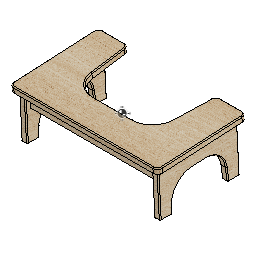
model (Autodesk Fusion 360 design; units mm, degrees)
Autodesk Fusion 360 part; units mm, degrees
sketch "top" plane through (0, 0, 0) normal (0, 0, 1) x (1, 0, 0) in component "stool"
  line L0 (0, 0) -> (500, 0)
  line L1 (120, 100.7611) -> (102.5689, 300)
  line L2 (102.5689, 300) -> (0, 300)
  line L3 (0, 300) -> (0, 0)
  line L4 (120, 100.7611) -> (380, 100.7611)
  line L5 (500, 300) -> (500, 0)
  line L6 (380, 100.7611) -> (397.4311, 300)
  line L7 (397.4311, 300) -> (500, 300)
  arc A0 (315.8568, 100.7611) -> (385.5904, 164.6602) centre (315.8568, 170.7611) ccw
  arc A1 (114.4096, 164.6602) -> (184.1432, 100.7611) centre (184.1432, 170.7611) ccw
  dimension "d5" = 300
  dimension "d6" = 500
  dimension "d7" = 260
  dimension "d8" = 200
  dimension "d21" = 70
  dimension "d36" = 95
  dimension "d37" = 95
  dimension "d42" = 294.8623
  dimension "d43" = 102.5689
  dimension "d44" = 100.7611
  constraint horizontal L0
  constraint horizontal L2
  constraint vertical L3
  constraint coincident L0.start L3.end
  constraint horizontal L4
  constraint vertical L5
  constraint horizontal L7
  constraint equal L2 L7
  constraint equal L3 L5
  constraint tangent L4 A0
  constraint coincident L4 A0.start
  constraint coincident L6 A0.end
  constraint tangent L1 A1
  constraint coincident L1 A1.start
  constraint coincident L4 A1.end
  constraint tangent L6 A0
  constraint tangent L4 A1
  constraint equal A0 A1
  measures "d5" distance of L0.start L2.end
  measures "d6" distance of L0.start L0.end
  measures "d7" distance of L1.start L4.end
  measures "d8" distance of L1.end L1.start
  measures "d21" radius of A0
  measures "d36" angle of L6 L7
  measures "d37" angle of L1 L2
  measures "d42" distance of L1.end L6.end
  measures "d43" distance of L6.end L5.start
  measures "d44" vertical distance of L0.end L4.end
extrude "Extrude1" add sketch "top" along normal blind 21 makes body 1 in component "stool"
move_body "Move1" bodies 1 to x (1, 0, 0) y (0, 0.99863, 0.052336) z (0, -0.052336, 0.99863) at (0, 1.8303, 0.0799) in component "stool"
sketch "side" plane through (0, 0, 0) normal (1, 0, 0) x (0, 1, 0) in component "stool"
  line L0 (285.4411, 14.9433) -> (294.0373, -149.0827)
  line L1 (294.0373, -149.0827) -> (254.0373, -149.0827)
  line L2 (254.0373, -149.0827) -> (247.5748, -103.0993)
  arc A0 (247.5748, -103.0993) -> (174.5925, -42.9374) centre (178.256, -112.8414) ccw
  line L3 (174.5925, -42.9374) -> (133.2386, -45.1046)
  arc A1 (133.2386, -45.1046) -> (66.9447, -112.5657) centre (136.9021, -115.0087) ccw
  line L4 (66.9447, -112.5657) -> (65.6695, -149.0827)
  line L5 (65.6695, -149.0827) -> (25.6695, -149.0827)
  line L6 (25.6695, -149.0827) -> (17.8083, 0.9173)
  line L7 (285.4411, 14.9433) -> (17.8083, 0.9173)
  line L8 (301.4191, 15.7807) -> (1.8303, 0.0799)
  dimension "d15" = 40
  dimension "d18" = 70
  dimension "d45" = 5
  dimension "d46" = 5
  dimension "d47" = 16
  dimension "d48" = 16
  dimension "d49" = 150
  dimension "d50" = 52
  constraint tangent L2 A0
  constraint tangent A0 L3
  constraint tangent L3 A1
  constraint tangent A1 L4
  constraint horizontal L5
  constraint equal L1 L5
  constraint equal A0 A1
  constraint perpendicular L6 L7
  constraint horizontal L1
  constraint perpendicular L0 L7
  constraint coincident L6.end L8
  constraint coincident L0.start L8
  constraint collinear L1 L5
  constraint parallel L3 L7
  measures "d15" distance of L0.end L1.end
  measures "d18" radius of A0
  measures "d45" angle of L0 L2
  measures "d46" angle of L4 L6
  measures "d47" distance of L0.start L8.start
  measures "d48" distance of L6.end L8.end
  measures "d49" vertical distance of L5.end L6.end
  measures "d50" distance of L3 L7
extrude "Extrude2" add sketch "side" along normal blind 21 from surface at 16 separate body makes body 2 in component "stool"
ref_plane "WorkPlane1" through (250, 151.0752, 18.4159) normal (-1, 0, 0) x (0, -0.99863, -0.052336) in component "stool"
mirror "Mirror1" about plane through (250, 151.0752, 18.4159) normal (-1, 0, 0) of bodies 2 makes body 3 in component "stool"
sketch "stretcher" plane through (37, 0, 0) normal (1, 0, 0) x (0, 1, 0) in component "stool"
  line L0 (294.0373, -149.0827) -> (285.4411, 14.9433)
  line L1 (285.4411, 14.9433) -> (17.8083, 0.9173)
  line L2 (17.8083, 0.9173) -> (25.6695, -149.0827)
  line L3 (25.6695, -149.0827) -> (65.6695, -149.0827)
  line L4 (65.6695, -149.0827) -> (66.9447, -112.5657)
  arc A0 (133.2386, -45.1046) -> (66.9447, -112.5657) centre (136.9021, -115.0087) ccw
  line L5 (133.2386, -45.1046) -> (174.5925, -42.9374)
  arc A1 (247.5748, -103.0993) -> (174.5925, -42.9374) centre (178.256, -112.8414) ccw
  line L6 (247.5748, -103.0993) -> (254.0373, -149.0827)
  line L7 (254.0373, -149.0827) -> (294.0373, -149.0827)
  line L8 (285.4411, 14.9433) -> (17.8083, 0.9173)
  line L9 (33.7864, 1.7547) -> (36.5079, -50.1741)
  line L10 (36.5079, -50.1741) -> (57.4791, -49.075)
  line L11 (57.4791, -49.075) -> (54.7576, 2.8537)
  dimension "d51" = 21
  dimension "d52" = 16
  dimension "d53" = 52
  constraint coincident L1 L9.start
  constraint coincident L1 L11.end
  constraint parallel L9 L11
  constraint perpendicular L1 L9
  constraint equal L9 L11
  measures "d51" distance of L9.end L10.end
  measures "d52" distance of L1.end L9.start
  measures "d53" distance of L9.start L9.end
extrude "Extrude4" add sketch "stretcher" along normal up to surface (426 mm away) separate body contours L1 L8 L9 L10 L11 makes body 4 in component "stool"
fillet "Fillet1" radius 16 6 edges at (0, 300.8696, 26.2663) (0, 1.2807, 10.5655) (500, 1.2807, 10.5655) (500, 300.8696, 26.2663) (102.5689, 300.8696, 26.2663) (397.4311, 300.8696, 26.2663) on bodies 1 in component "stool"
fillet "Fillet2" radius 3.175 30 edges at (16, 250.806, -126.091) (16, 222.7815, -58.8277) (16, 153.9155, -44.021) (16, 86.9745, -65.9451) (16, 66.3071, -130.8242) (16, 21.7389, -74.0827) (37, 21.7389, -74.0827) (37, 289.7392, -67.0697) (16, 289.7392, -67.0697) (37, 66.3071, -130.8242) (37, 86.9745, -65.9451) (37, 153.9155, -44.021) (37, 222.7815, -58.8277) (37, 250.806, -126.091) (463, 66.3071, -130.8242) (463, 86.9745, -65.9451) (463, 153.9155, -44.021) (463, 222.7815, -58.8277) (463, 250.806, -126.091) (484, 250.806, -126.091) (484, 222.7815, -58.8277) (484, 153.9155, -44.021) (484, 86.9745, -65.9451) (484, 66.3071, -130.8242) (463, 21.7389, -74.0827) (484, 21.7389, -74.0827) (484, 289.7392, -67.0697) (463, 289.7392, -67.0697) (250, 36.5079, -50.1741) (250, 57.4791, -49.075) 6 faces at (461.8635, 155.4057, 29.1573) (461.8635, 156.5047, 8.1861) (23, 280.704, -149.0827) (23, 52.3362, -149.0827) (477, 280.704, -149.0827) (477, 39.0028, -149.0827) on bodies 1 2 3 4 in component "stool"
component "stool" placed x (1, 0, 0) y (0, 1, 0) z (0, 0, 1) at (0, 0, 0)
equation "width = 500 mm"
equation "depth = 300 mm"
equation "holeWidth = 260 mm"
equation "holeDepth = 200 mm"
equation "d5 = depth"
equation "d6 = width"
equation "d7 = holeWidth"
equation "d8 = holeDepth"
equation "thickness = 21 mm"
equation "d10 = thickness"
equation "inset = 16 mm"
equation "d15 = memberWidth"
equation "height = 150 mm"
equation "d18 = largeRadius"
equation "memberWidth = 40 mm"
equation "largeRadius = 70 mm"
equation "d21 = largeRadius"
equation "d22 = inset"
equation "d23 = thickness"
equation "stretcherWidth = memberWidth * 1.3"
equation "taper = 5 deg"
equation "d36 = 90 deg + taper"
equation "d37 = 90 deg + taper"
equation "d39 = inset"
equation "d41 = 1/8\""
equation "d45 = taper"
equation "d46 = taper"
equation "d47 = inset"
equation "d48 = inset"
equation "d49 = height"
equation "d50 = stretcherWidth"
equation "d51 = thickness"
equation "d52 = inset"
equation "d53 = stretcherWidth"
